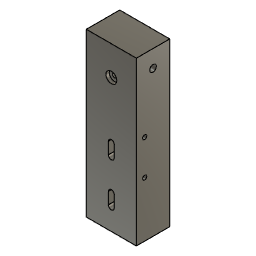
test v1 (Autodesk Fusion 360 design; units mm, degrees)
Autodesk Fusion 360 part; units mm, degrees
sketch "Skizze1" plane through (0, 0, 0) normal (0, 0, 1) x (1, 0, 0)
  line L0 (30, 20) -> (-30, 20)
  line L1 (-30, 20) -> (-30, -20)
  line L2 (-30, -20) -> (30, -20)
  line L3 (30, -20) -> (30, 20)
  line L4 (30, 20) -> (-30, -20) construction
  line L5 (-30, 20) -> (30, -20) construction
  dimension "d2" = 60
  dimension "d3" = 40
  constraint perpendicular L0 L1
  constraint parallel L0 L2
  constraint parallel L1 L3
  constraint horizontal L0
  constraint coincident L4 origin
  constraint coincident L5 origin
  measures "d2" distance of L1.end L2.end
  measures "d3" distance of L0.end L1.end
extrude "Extrusion1" add sketch "Skizze1" along normal blind 195
sketch "Skizze3" plane through (0, -20, 0) normal (0, -1, 0) x (1, 0, 0)
  line L0 (-30, 0) -> (30, 0)
  line L1 (30, 0) -> (30, 195)
  line L2 (30, 195) -> (-30, 195)
  line L3 (-30, 195) -> (-30, 0)
  line L4 (-3.5, 40) -> (-3.5, 26)
  arc A0 (-3.5, 26) -> (3.5, 26) centre (0, 26) ccw
  line L5 (3.5, 26) -> (3.5, 40)
  arc A1 (3.5, 40) -> (-3.5, 40) centre (0, 40) ccw
  line L6 (0, 40) -> (0, 26) construction
  line L7 (-3.5, 92) -> (-3.5, 78)
  arc A2 (-3.5, 78) -> (3.5, 78) centre (0, 78) ccw
  line L8 (3.5, 78) -> (3.5, 92)
  arc A3 (3.5, 92) -> (-3.5, 92) centre (0, 92) ccw
  line L9 (0, 92) -> (0, 78) construction
  point P0 (0, 195)
  dimension "d6" = 14
  dimension "d7" = 7
  dimension "d8" = 14
  dimension "d9" = 7
  constraint tangent L4 A0
  constraint tangent A0 L5
  constraint parallel L4 L5
  constraint tangent L5 A1
  constraint tangent L4 A1
  constraint vertical L6
  constraint midpoint L2 P0
  constraint vertical A1.centre P0
  constraint tangent L7 A2
  constraint tangent A2 L8
  constraint parallel L7 L8
  constraint tangent L8 A3
  constraint tangent L7 A3
  constraint vertical L9
  constraint vertical P0 A3.centre
  measures "d6" distance of A1.centre A0.centre
  measures "d7" diameter of A0
  measures "d8" distance of A3.centre A2.centre
  measures "d9" diameter of A2
extrude "Extrusion2" cut sketch "Skizze3" against normal blind 40 contours L4 A0 L5 A1 | L7 A2 L8 A3
sketch "Skizze4" plane through (30, 0, 0) normal (1, 0, 0) x (0, 1, 0)
  line L0 (-20, 0) -> (20, 0)
  line L1 (20, 0) -> (20, 195)
  line L2 (20, 195) -> (-20, 195)
  line L3 (-20, 195) -> (-20, 0)
  circle A0 centre (0, 174.5) radius 4
  dimension "d12" = 8
  measures "d12" diameter of A0
extrude "Extrusion3" cut sketch "Skizze4" against normal blind 60 contours A0
sketch "Skizze6" plane through (0, 0, 0) normal (0, 1, 0) x (1, 0, 0)
sketch "Skizze7" plane through (0, 20, 0) normal (0, 1, 0) x (-1, 0, 0)
  line L0 (3.5, 40) -> (3.5, 26)
  arc A0 (-3.5, 26) -> (3.5, 26) centre (0, 26) ccw
  line L1 (-3.5, 26) -> (-3.5, 40)
  arc A1 (3.5, 40) -> (-3.5, 40) centre (0, 40) ccw
  line L2 (3.5, 92) -> (3.5, 78)
  arc A2 (-3.5, 78) -> (3.5, 78) centre (0, 78) ccw
  line L3 (-3.5, 78) -> (-3.5, 92)
  arc A3 (3.5, 92) -> (-3.5, 92) centre (0, 92) ccw
  line L4 (-30, 0) -> (30, 0)
  line L5 (30, 0) -> (30, 195)
  line L6 (30, 195) -> (-30, 195)
  line L7 (-30, 195) -> (-30, 0)
  circle A4 centre (0, 160) radius 2.5
  dimension "d17" = 5
  measures "d17" diameter of A4
extrude "Extrusion4" cut sketch "Skizze7" against normal blind 40 contours A4
sketch "Skizze9" plane through (30, 0, 0) normal (1, 0, 0) x (0, 1, 0)
  circle A0 centre (0, 174.5) radius 4
  line L0 (-20, 0) -> (20, 0)
  line L1 (20, 0) -> (20, 195)
  line L2 (20, 195) -> (-20, 195)
  line L3 (-20, 195) -> (-20, 0)
  circle A1 centre (-10, 108) radius 2.5
  circle A2 centre (-10, 66) radius 2.5
  dimension "d23" = 5
  dimension "d24" = 5
  measures "d23" diameter of A1
  measures "d24" diameter of A2
extrude "Extrusion6" cut sketch "Skizze9" against normal blind 80 contours A1 | A2
sketch "Skizze10" plane through (0, 20, 0) normal (0, 1, 0) x (-1, 0, 0)
  circle A0 centre (0, 160) radius 2.5
  line L0 (3.5, 40) -> (3.5, 26)
  arc A1 (-3.5, 26) -> (3.5, 26) centre (0, 26) ccw
  line L1 (-3.5, 26) -> (-3.5, 40)
  arc A2 (3.5, 40) -> (-3.5, 40) centre (0, 40) ccw
  line L2 (3.5, 92) -> (3.5, 78)
  arc A3 (-3.5, 78) -> (3.5, 78) centre (0, 78) ccw
  line L3 (-3.5, 78) -> (-3.5, 92)
  arc A4 (3.5, 92) -> (-3.5, 92) centre (0, 92) ccw
  line L4 (-30, 0) -> (30, 0)
  line L5 (30, 0) -> (30, 195)
  line L6 (30, 195) -> (-30, 195)
  line L7 (-30, 195) -> (-30, 0)
  circle A5 centre (0, 160) radius 6.5
  dimension "d27" = 13
  constraint concentric A0 A5
  measures "d27" diameter of A5
extrude "Extrusion7" cut sketch "Skizze10" against normal blind 4 contours A5
sketch "Skizze11" plane through (0, -20, 0) normal (0, -1, 0) x (1, 0, 0)
  circle A0 centre (0, 160) radius 2.5
  line L0 (-3.5, 26) -> (-3.5, 40)
  arc A1 (3.5, 40) -> (-3.5, 40) centre (0, 40) ccw
  line L1 (3.5, 40) -> (3.5, 26)
  arc A2 (-3.5, 26) -> (3.5, 26) centre (0, 26) ccw
  line L2 (-3.5, 78) -> (-3.5, 92)
  arc A3 (3.5, 92) -> (-3.5, 92) centre (0, 92) ccw
  line L3 (3.5, 92) -> (3.5, 78)
  arc A4 (-3.5, 78) -> (3.5, 78) centre (0, 78) ccw
  line L4 (-30, 0) -> (30, 0)
  line L5 (30, 0) -> (30, 195)
  line L6 (30, 195) -> (-30, 195)
  line L7 (-30, 195) -> (-30, 0)
  circle A5 centre (0, 160) radius 6.5
  dimension "d30" = 13
  constraint concentric A0 A5
  measures "d30" diameter of A5
extrude "Extrusion8" cut sketch "Skizze11" against normal blind 4 contours A5
